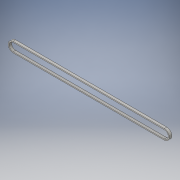
# Autodesk Inventor part: 16inchliftwire
Saved by Autodesk Inventor 2016 (Build 200138000, 138)
## iProperties
Created: 2017-01-16
Part Number: 16inchliftwire
Material: Generic
Document SubType Name: Modeling
Designer: RoboticsUser
Density: 1 g/cm^3
Appearance: Default
Author: RoboticsUser
Autodesk Inventor part; units mm, degrees
ref_plane "YZ Plane" through (0, 0, 0) normal (1, 0, 0) x (0, 1, 0)
ref_plane "XZ Plane" through (0, 0, 0) normal (0, 1, 0) x (-1, 0, 0)
ref_plane "XY Plane" through (0, 0, 0) normal (0, 0, 1) x (1, 0, 0)
sketch "Sketch1" plane through (0, 0, 0) normal (0, 0, 1) x (1, 0, 0)
  line L0 (0, 0) -> (406.4, 0)
  line L1 (406.4, 0) -> (406.4, 25.4)
  line L2 (406.4, 25.4) -> (0, 25.4)
  line L3 (0, 25.4) -> (0, 0)
  dimension "d0" = 406.4
  dimension "d1" = 25.4
  constraints: 8 end point, 2 parallel, 1 horizontal, 1 perpendicular
  measures "d0" distance of L2.end L1.end
  measures "d1" distance of L1.end L0.end
extrude "Extrusion1" add sketch "Sketch1" along normal blind 6.35
fillet "Fillet1" radius 12.7 1 edges at (406.4, 25.4, 3.175)
fillet "Fillet2" radius 12.7 1 edges at (406.4, 0, 3.175)
fillet "Fillet3" radius 12.7 1 edges at (0, 25.4, 3.175)
fillet "Fillet4" radius 12.7 1 edges at (0, 0, 3.175)
shell "Shell1" thickness 2.54 removed faces 2 at (266.7, 8.4667, 6.35) at (266.7, 8.4667, 0)
body "Solid1"
